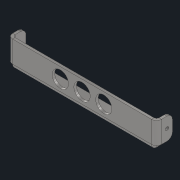
# Autodesk Inventor part: plate2
Saved by Autodesk Inventor 2021 (Build 250183000, 183)
## iProperties
Created: 2021-07-19
Part Number: plate2
Material: 鋼、炭素鋼
Document SubType Name: Sheet Metal
Designer: yuta0
Density: 7.85 g/cm^3
Sheet Metal Rule: Default_mm
Appearance: 半つや出し
Mass: 110.749 g
Surface Area: 134.224 cm^2
Volume: 14.1082 cm^3
Author: yuta0
Autodesk Inventor part; units mm, degrees
ref_plane "YZ Plane" through (0, 0, 0) normal (1, 0, 0) x (0, 1, 0)
ref_plane "XZ Plane" through (0, 0, 0) normal (0, 1, 0) x (-1, 0, 0)
ref_plane "XY Plane" through (0, 0, 0) normal (0, 0, 1) x (1, 0, 0)
sketch "スケッチ1" plane through (0, 0, 0) normal (0, 0, 1) x (1, 0, 0)
  line L0 (-68.5, -10) -> (68.5, -10)
  line L1 (68.5, -10) -> (68.5, 10)
  line L2 (68.5, 10) -> (-68.5, 10)
  line L3 (-68.5, 10) -> (-68.5, -10)
  line L4 (-68.5, -10) -> (68.5, 10) construction
  line L5 (68.5, -10) -> (-68.5, 10) construction
  point P0 (0, 0)
  dimension "d0" = 20
  dimension "d1" = 137
  measures "d0" distance of L0.end L1.end
  measures "d1" distance of L1.end L2.end
extrude "プレート1" add sketch "スケッチ1" along normal blind 2.3
sketch "スケッチ2" plane through (66.2, -10, 2.3) normal (1, 0, 0) x (0, 1, 0)
  line L0 (20, 0) -> (0, 0)
  line L1 (0, 0) -> (0, -14.6)
  line L2 (0, -14.6) -> (20, -14.6)
  line L3 (20, -14.6) -> (20, 0)
  constraints: 6 end point, 1 horizontal, 1 perpendicular, 1 vertical
edge flange "フランジ1" height 14.6 angle 90 thickness 2.3 bend radius 2.3 thickness toward (1, 0, 0) relief tear relief width 2.3 relief depth 1.15 corner gap 2.3 corner form 0 edges at (68.5, 0, 0) (-68.5, 0, 0) wall of the first edge with corners at (66.2, 10, 2.3) (66.2, -10, 2.3) (66.2, -10, -12.3) (66.2, 10, -12.3)
bend "曲げ1"
corner "コーナー1"
sketch "スケッチ7" plane through (-63.9, -12.3, -2.3) normal (0, -1, 0) x (1, 0, 0)
  line L0 (127.8, 0) -> (0, 0)
  line L1 (0, 0) -> (0, -10)
  line L2 (0, -10) -> (127.8, -10)
  line L3 (127.8, -10) -> (127.8, 0)
  constraints: 6 end point, 1 horizontal, 1 perpendicular, 1 vertical
edge flange "フランジ2" height 14.6 angle 90 thickness 2.3 bend radius 2.3 thickness toward (0, -1, 0) relief tear relief width 2.3 relief depth 1.15 edges at (0, -10, 0) wall of the first edge with corners at (63.9, -12.3, -2.3) (-63.9, -12.3, -2.3) (-63.9, -12.3, -12.3) (63.9, -12.3, -12.3)
bend "曲げ2"
corner "コーナー2"
sketch "スケッチ5" plane through (68.5, -10, -12.3) normal (1, 0, 0) x (0, 0, -1)
  line L0 (-10, 20) -> (0, 20) projected
  line L1 (0, 20) -> (0, 0) projected
  line L2 (-10, -4.6) -> (0, -4.6) projected
  line L3 (0, 0) -> (-10, 0) projected
  point P0 (-12.3, 10)
  point P1 (-5, 25.4)
  point P2 (-5, 10)
  dimension "d80" = 5
  dimension "d95" = 30
  dimension "d106" = 10
  constraints: 1 vertical alignment
  measures "d80" distance from line of L1 point (-5, 25.4)
  measures "d95" distance from line of point (-5, 25.4) L2
  measures "d106" distance from line of point (-5, 10) L3
hole "穴3" at (68.5, 15.4, -7.3) at (68.5, 0, -7.3) direction (-1, 0, 0) diameter 3.242 end through all thread size "M4x0.7" class "6H" standard "ANSI Metric M Profile"
sketch "スケッチ9" plane through (-63.9, -14.6, -12.3) normal (0, -1, 0) x (1, 0, 0)
  line L0 (127.8, 0) -> (0, 0) projected
  line L1 (0, 0) -> (0, 10) projected
  line L2 (127.8, 10) -> (127.8, 0) projected
  point P0 (63.9, 12.3)
  point P1 (122.8, 5)
  point P2 (5, 5)
  dimension "d82" = 5
  dimension "d83" = 5
  dimension "d84" = 5
  constraints: 1 horizontal alignment
  measures "d82" distance from line of L0 point (5, 5)
  measures "d83" distance from line of L1 point (5, 5)
  measures "d84" distance from line of L2 point (122.8, 5)
hole "穴5" at (58.9, -14.6, -7.3) at (-58.9, -14.6, -7.3) direction (0, 1, 0) diameter 3.4 end through all clearance for "Flat Head Machine Screw" size "M3" standard "Ansi Metric M Profile"
fillet "コーナーR2" radius 5 6 edges at (67.35, 10, -12.3) (63.9, -13.45, -12.3) (-63.9, -13.45, -12.3) (-67.35, 10, -12.3) (67.35, -10, -12.3) (-67.35, -10, -12.3)
sketch "スケッチ10" plane through (0, 0, 2.3) normal (0, 0, 1) x (1, 0, 0)
  circle A0 centre (0, 0) radius 7.5
  circle A1 centre (-20, 0) radius 7.5
  circle A2 centre (20, 0) radius 7.5
  dimension "d96" = 15
  dimension "d99" = 15
  dimension "d101" = 15
  dimension "d104" = 20
  dimension "d107" = 20
  constraints: 3 centre point, 2 coincident, 2 horizontal alignment
  measures "d96" diameter of A0
  measures "d99" diameter of A1
  measures "d101" diameter of A2
  measures "d104" distance of A1.centre A0.centre
  measures "d107" distance of A2.centre A0.centre
extrude "押し出し2" cut sketch "スケッチ10" against normal blind 10
equation "\"d48\" = Thickness"
equation "\"d90\" = Thickness"
equation "\"d2\" = Thickness"
equation "\"d3\" = BendReliefWidth"
equation "\"d4\" = BendReliefDepth"
equation "\"d5\" = MinimumRemnant"
equation "\"d6\" = TransitionRadius"
equation "\"d9\" = BendRadius"
equation "\"d10\" = CornerReliefSize"
equation "\"d11\" = GapSize"
equation "\"d12\" = JacobiRadiusSize"
equation "\"d68\" = BendReliefWidth"
equation "\"d69\" = BendReliefDepth"
equation "\"d70\" = MinimumRemnant"
equation "\"d71\" = TransitionRadius"
equation "\"d74\" = BendRadius"
equation "\"d75\" = CornerReliefSize"
equation "\"d76\" = GapSize"
equation "\"d77\" = JacobiRadiusSize"
equation "\"BendRadius\" = Thickness"
equation "\"BendReliefWidth\" = Thickness"
equation "\"BendReliefDepth\" = 0.5 * Thickness"
equation "\"CornerReliefSize\" = 4 * Thickness"
equation "\"MinimumRemnant\" = 2 * Thickness"
equation "\"TransitionRadius\" = BendRadius"
equation "\"JacobiRadiusSize\" = BendRadius"
equation "\"GapSize\" = Thickness"
equation "\"Thickness\" = 2.3"
